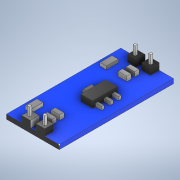
# Autodesk Inventor part: dc to dc
Saved by Autodesk Inventor 2021 (Build 250183000, 183)
## iProperties
Created: 2021-07-15
Part Number: dc to dc
Material: Generic
Document SubType Name: Modeling
Designer: HP
Density: 1 g/cm^3
Appearance: Default
Author: HP
Autodesk Inventor part; units mm, degrees
ref_plane "YZ Plane" through (0, 0, 0) normal (1, 0, 0) x (0, 1, 0)
ref_plane "XZ Plane" through (0, 0, 0) normal (0, 1, 0) x (-1, 0, 0)
ref_plane "XY Plane" through (0, 0, 0) normal (0, 0, 1) x (1, 0, 0)
sketch "Sketch1" plane through (0, 0, 0) normal (0, 1, 0) x (-1, 0, 0)
  line L0 (0, 0) -> (12, 0)
  line L1 (12, 0) -> (12, -26)
  line L2 (12, -26) -> (0, -26)
  line L3 (0, -26) -> (0, 0)
  dimension "d0" = 12
  dimension "d1" = 26
  constraints: 8 end point, 2 parallel, 1 horizontal, 1 perpendicular
  measures "d0" distance of L1.end L2.end
  measures "d1" distance of L0.end L1.end
extrude "Extrusion1" add sketch "Sketch1" along normal blind 1
sketch "Sketch2" plane through (0, 1, 0) normal (0, 1, 0) x (1, 0, 0)
  line L0 (-8.4967, 0) -> (-6.4967, 0)
  line L1 (-6.4967, 0) -> (-6.4967, 2)
  line L2 (-6.4967, 2) -> (-8.4967, 2)
  line L3 (-8.4967, 2) -> (-8.4967, 0)
  line L4 (-5.264, 0) -> (-3.264, 0)
  line L5 (-3.264, 0) -> (-3.264, 2)
  line L6 (-3.264, 2) -> (-5.264, 2)
  line L7 (-5.264, 2) -> (-5.264, 0)
  line L8 (0, 26) -> (-12, 26) projected
  line L9 (-8.4967, 26) -> (-6.4967, 26)
  line L10 (-6.4967, 26) -> (-6.4967, 24)
  line L11 (-6.4967, 24) -> (-8.4967, 24)
  line L12 (-8.4967, 24) -> (-8.4967, 26)
  line L13 (-5.264, 24) -> (-3.264, 24)
  line L14 (-3.264, 24) -> (-3.264, 26)
  line L15 (-3.264, 26) -> (-5.264, 26)
  line L16 (-5.264, 26) -> (-5.264, 24)
  line L17 (-6, 10.9212) -> (-3.3419, 10.9212)
  line L18 (-3.3419, 10.9212) -> (-3.3419, 16.5565)
  line L19 (-3.3419, 16.5565) -> (-6, 16.5565)
  line L20 (-6, 16.5565) -> (-6, 10.9212)
  point P0 (0, 0)
  dimension "d4" = 2
  dimension "d5" = 2
  dimension "d6" = 2
  dimension "d7" = 2
  dimension "d8" = 2
  constraints: 40 end point, 10 parallel, 8 point on line, 5 horizontal, 5 perpendicular
  measures "d4" distance of L2.end L1.end
  measures "d5" distance of L1.end L0.end
  measures "d6" distance of L6.end L5.end
  measures "d7" distance of L10.end L11.end
  measures "d8" distance of L9.end L10.end
extrude "Extrusion2" add sketch "Sketch2" along normal blind 1.5
sketch "Sketch3" plane through (0, 2.5, 0) normal (0, 1, 0) x (1, 0, 0)
  line L0 (-7.7977, 0.5679) -> (-7.2977, 0.5679)
  line L1 (-7.2977, 0.5679) -> (-7.2977, 1.0679)
  line L2 (-7.2977, 1.0679) -> (-7.7977, 1.0679)
  line L3 (-7.7977, 1.0679) -> (-7.7977, 0.5679)
  line L4 (-4.303, 0.5679) -> (-3.803, 0.5679)
  line L5 (-3.803, 0.5679) -> (-3.803, 1.0679)
  line L6 (-3.803, 1.0679) -> (-4.303, 1.0679)
  line L7 (-4.303, 1.0679) -> (-4.303, 0.5679)
  line L8 (-7.7977, 24.5946) -> (-7.2977, 24.5946)
  line L9 (-7.2977, 24.5946) -> (-7.2977, 25.0946)
  line L10 (-7.2977, 25.0946) -> (-7.7977, 25.0946)
  line L11 (-7.7977, 25.0946) -> (-7.7977, 24.5946)
  line L12 (-4.303, 24.5946) -> (-3.803, 24.5946)
  line L13 (-3.803, 24.5946) -> (-3.803, 25.0946)
  line L14 (-3.803, 25.0946) -> (-4.303, 25.0946)
  line L15 (-4.303, 25.0946) -> (-4.303, 24.5946)
  point P0 (0, 0)
  dimension "d11" = 0.5
  dimension "d12" = 0.5
  dimension "d13" = 0.5
  dimension "d14" = 0.5
  dimension "d15" = 0.5
  dimension "d16" = 0.5
  constraints: 32 end point, 8 parallel, 6 point on line, 4 horizontal, 4 perpendicular
  measures "d11" distance of L2.end L1.end
  measures "d12" distance of L1.end L0.end
  measures "d13" distance of L6.end L5.end
  measures "d14" distance of L10.end L9.end
  measures "d15" distance of L9.end L8.end
  measures "d16" distance of L14.end L13.end
extrude "Extrusion3" add sketch "Sketch3" along normal blind 2
sketch "Sketch4" plane through (0, 1, 0) normal (0, 1, 0) x (1, 0, 0)
  line L0 (-6.7275, 22.8918) -> (-4.7275, 22.8918)
  line L1 (-4.7275, 22.8918) -> (-4.7275, 21.8918)
  line L2 (-4.7275, 21.8918) -> (-6.7275, 21.8918)
  line L3 (-6.7275, 21.8918) -> (-6.7275, 22.8918)
  line L4 (-6.7275, 20.1179) -> (-4.7275, 20.1179)
  line L5 (-4.7275, 20.1179) -> (-4.7275, 21.1179)
  line L6 (-4.7275, 21.1179) -> (-6.7275, 21.1179)
  line L7 (-6.7275, 21.1179) -> (-6.7275, 20.1179)
  line L8 (-4.7275, 4.0841) -> (-6.7275, 4.0841)
  line L9 (-6.7275, 4.0841) -> (-6.7275, 3.0841)
  line L10 (-6.7275, 3.0841) -> (-4.7275, 3.0841)
  line L11 (-4.7275, 3.0841) -> (-4.7275, 4.0841)
  line L12 (-6.7275, 4.8554) -> (-4.7275, 4.8554)
  line L13 (-4.7275, 4.8554) -> (-4.7275, 5.8554)
  line L14 (-4.7275, 5.8554) -> (-6.7275, 5.8554)
  line L15 (-6.7275, 5.8554) -> (-6.7275, 4.8554)
  point P0 (0, 0)
  dimension "d19" = 2
  dimension "d20" = 1
  dimension "d21" = 2
  dimension "d22" = 1
  dimension "d23" = 2
  dimension "d24" = 1
  dimension "d25" = 2
  dimension "d26" = 1
  constraints: 32 end point, 8 parallel, 4 horizontal, 4 perpendicular, 1 point on line
  measures "d19" distance of L1.end L2.end
  measures "d20" distance of L0.end L1.end
  measures "d21" distance of L6.end L5.end
  measures "d22" distance of L5.end L4.end
  measures "d23" distance of L10.end L9.end
  measures "d24" distance of L9.end L8.end
  measures "d25" distance of L14.end L13.end
  measures "d26" distance of L13.end L12.end
extrude "Extrusion4" add sketch "Sketch4" along normal blind 1
sketch "Sketch5" plane through (0, 1, 0) normal (0, 1, 0) x (1, 0, 0)
  line L0 (-10.8338, 5.7882) -> (-9.3922, 5.7882)
  line L1 (-9.3922, 5.7882) -> (-9.3922, 3.0841)
  line L2 (-9.3922, 3.0841) -> (-10.8338, 3.0841)
  line L3 (-10.8338, 3.0841) -> (-10.8338, 5.7882)
  line L4 (-10.8338, 22.8302) -> (-9.3922, 22.8302)
  line L5 (-9.3922, 22.8302) -> (-9.3922, 20.0926)
  line L6 (-9.3922, 20.0926) -> (-10.8338, 20.0926)
  line L7 (-10.8338, 20.0926) -> (-10.8338, 22.8302)
  point P0 (0, 0)
  constraints: 16 end point, 4 parallel, 2 horizontal, 2 perpendicular, 2 point on line
extrude "Extrusion5" add sketch "Sketch5" along normal blind 0.7
sketch "Sketch6" plane through (0, 1, 0) normal (0, 1, 0) x (1, 0, 0)
  point P0 (0, 0)
sketch "Sketch7" plane through (0, 1, 0) normal (0, 1, 0) x (1, 0, 0)
  line L0 (-3.3419, 16.5565) -> (-3.3419, 10.9212) projected
  line L1 (-3.3419, 16.0376) -> (-1.9546, 16.0376)
  line L2 (-1.9546, 16.0376) -> (-1.9546, 15.4008)
  line L3 (-1.9546, 15.4008) -> (-3.3419, 15.4008)
  line L4 (-3.3419, 15.4008) -> (-3.3419, 16.0376)
  line L5 (-3.3419, 14.1925) -> (-1.9546, 14.1925)
  line L6 (-1.9546, 14.1925) -> (-1.9546, 13.5115)
  line L7 (-1.9546, 13.5115) -> (-3.3419, 13.5115)
  line L8 (-3.3419, 13.5115) -> (-3.3419, 14.1925)
  line L9 (-3.3419, 12.1636) -> (-1.9546, 12.1636)
  line L10 (-1.9546, 12.1636) -> (-1.9546, 11.5661)
  line L11 (-1.9546, 11.5661) -> (-3.3419, 11.5661)
  line L12 (-3.3419, 11.5661) -> (-3.3419, 12.1636)
  line L13 (-6, 10.9212) -> (-6, 16.5565) projected
  line L14 (-6, 14.8304) -> (-7.4823, 14.8304)
  line L15 (-7.4823, 14.8304) -> (-7.4823, 12.8104)
  line L16 (-7.4823, 12.8104) -> (-6, 12.8104)
  line L17 (-6, 12.8104) -> (-6, 14.8304)
  point P0 (0, 0)
  constraints: 32 end point, 8 parallel, 6 point on line, 4 horizontal, 4 perpendicular
extrude "Extrusion6" add sketch "Sketch7" along normal blind 0.7
body "Solid1"
